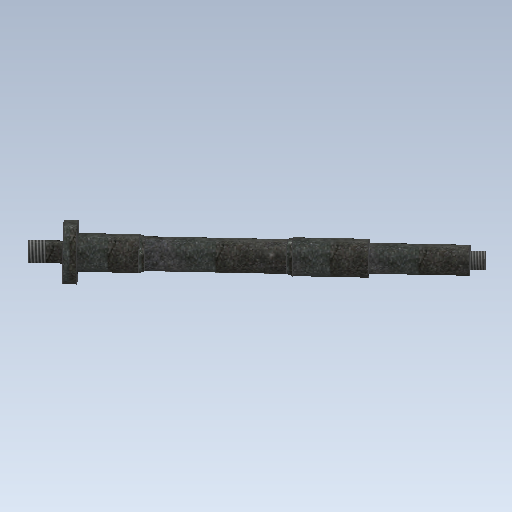
# Autodesk Inventor part: DEC_tengely
Saved by Autodesk Inventor 2021.4 (Build 254397000, 397)
## iProperties
Created: 2023-11-18
Part Number: DEC_tengely
Material: Steel
Document SubType Name: Modeling
Designer: vtoth
Density: 7.85 g/cm^3
Appearance: Plate
Mass: 484.272 g
Surface Area: 149.467 cm^2
Volume: 61.6907 cm^3
Author: vtoth
Autodesk Inventor part; units mm, degrees
ref_plane "YZ Plane" through (0, 0, 0) normal (1, 0, 0) x (0, 1, 0)
ref_plane "XZ Plane" through (0, 0, 0) normal (0, 1, 0) x (-1, 0, 0)
derived "skeleton_1.ipt"
sketch "Sketch1" plane through (0, 0, 0) normal (0, 1, 0) x (-1, 0, 0)
  line L0 (0, 0) -> (0, 550)
  circle A0 centre (0, 550) radius 6
  line L1 (0, 550) -> (43.8812, 590.9199)
  line L2 (-15.7936, 654.9134) -> (83.0961, 548.8671)
  line L3 (111.4949, 533.0759) -> (80.291, 566.538)
  line L4 (96.8679, 519.4359) -> (65.6639, 552.898)
  line L5 (0, 0) -> (-350, 0)
  line L6 (11.0017, 632.044) -> (5.1509, 626.588)
  point P0 (0, 440)
sketch "Sketch2" plane through (15.7936, 0, 654.9134) normal (-0.6819984, 0, -0.7313537) x (0, -1, 0)
  line L0 (0, -60) -> (0, 0) construction
  line L1 (0, -72) -> (0, 80)
  circle A0 centre (0, 0) radius 10
  line L2 (10, -4.956) -> (10, -4.9245)
  line L3 (-10, 4.9268) -> (-10, 4.959)
  line L4 (-5, 73) -> (5, 73)
  point P0 (0, 0)
  point P1 (0, 0)
  point P2 (0, 0)
  point P3 (0, 10)
  point P4 (0, 10)
  point P5 (0, 10)
  point P6 (0, -57)
  point P7 (0, 45)
sketch "Sketch3" plane through (-42.7147, 0, 709.4732) normal (-0.7313537, 0, 0.6819984) x (0, -1, 0)
  line L0 (0, 0) -> (0, -145) construction
  line L1 (105, 0) -> (-105, 0)
  circle A0 centre (0, 0) radius 6
  line L2 (0, 50) -> (0, -50)
  line L3 (-105, -80) -> (-105, 80)
  point P0 (0, 0)
  point P1 (0, 0)
  point P2 (0, 0)
  point P3 (0, 0)
  point P4 (-79, -23)
ref_plane "Work Plane1" through (15.7936, 0, 654.9134) normal (-0.6819984, 0, -0.7313537) x (0, -1, 0)
ref_plane "Work Plane2" through (-42.7147, 0, 709.4732) normal (-0.7313537, 0, 0.6819984) x (0, -1, 0)
ref_plane "Work Plane3" through (68.4511, 0, 605.8095) normal (0.6819984, 0, 0.7313537) x (-0.7313537, 0, 0.6819984)
sketch "Sketch4" plane through (68.4511, 0, 605.8095) normal (0.6819984, 0, 0.7313537) x (-0.7313537, 0, 0.6819984)
  line L0 (0, 0) -> (152, 0) construction
  line L1 (145, -5) -> (145, 5) construction
  line L2 (152, -6) -> (152, 6) construction
  line L3 (170, 0) -> (170, -6)
  line L4 (170, -6) -> (152, -6)
  line L5 (152, -6) -> (152, -16.5)
  line L6 (152, -16.5) -> (145, -16.5)
  line L7 (145, -16.5) -> (145, -10)
  line L8 (145, -10) -> (113, -10)
  line L9 (113, -10) -> (110, -9)
  line L10 (110, -9) -> (37, -9)
  line L11 (37, -9) -> (34, -10)
  line L12 (34, -10) -> (-5, -10)
  line L13 (-5, -10) -> (-5, -8)
  line L14 (-5, -8) -> (-57, -8)
  line L15 (-57, -8) -> (-57, -5)
  line L16 (-57, -5) -> (-65, -5)
  line L17 (-65, -5) -> (-65, 0)
  line L18 (73.5, -82.7302) -> (73.5, -74.2698) construction
  line L19 (-65, 0) -> (170, 0)
  line L20 (76.9268, -10) -> (76.959, -10) projected
  point P0 (-363.0991, 0)
  dimension "d1" = 18
  dimension "d2" = 150
  dimension "d3" = 52
  dimension "d5" = 33
  dimension "d6" = 12
  dimension "d7" = 18
  dimension "d8" = 32
  dimension "d9" = 39
  dimension "d11" = 73
  dimension "d12" = 16
  dimension "d13" = 10
  dimension "d14" = 8
  constraints: 34 end point, 10 perpendicular, 5 point on line, 3 collinear, 2 symmetric about line, 1 parallel
  measures "d1" diameter of L10 L0
  measures "d2" distance between parallel lines of L13 L7
  measures "d3" distance between parallel lines of L15 L13
  measures "d5" diameter of L6 L0
  measures "d6" diameter of L4 L0
  measures "d7" distance between parallel lines of L5 L3
  measures "d8" distance of L8.end L7.end
  measures "d9" distance from line of L13 L11.end
  measures "d11" distance of L10.end L9.end
  measures "d12" diameter of L14 L0
  measures "d13" diameter of L16 L0
  measures "d14" distance between parallel lines of L15 L17
revolve "Revolution1" add sketch "Sketch4" angle 360 about axis through (68.4511, 0, 605.8095) along (-0.7313537, 0, 0.6819984)
sketch "Sketch5" plane through (-42.7147, 0, 709.4732) normal (-0.7313537, 0, 0.6819984) x (-0.6819984, 0, -0.7313537)
  circle A0 centre (0, 0) radius 6 projected
  circle A1 centre (0, 0) radius 7
  circle A2 centre (0, 0) radius 25
  point P0 (489.7445, 0)
  dimension "d16" = 50
  dimension "d17" = 1
  constraints: 2 centre point, 2 coincident
  measures "d16" diameter of A2
  measures "d17" radial gap between concentric circles of A0 A1
extrude "Extrusion1" [suppressed]
thread "Thread1" size "M10x1.5" class "6g" standard "ISO Metric profile" full length
thread "Thread2" size "M12x1.75" class "6g" standard "ANSI Metric M Profile" length 9
body "Solid1"
